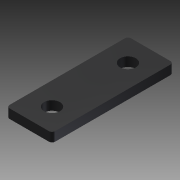
# Autodesk Inventor part: D-023
Saved by Autodesk Inventor 2015 (Build 190159000, 159)
## iProperties
Company: MARCHA TECHNOLOGY
Created: 2014-01-21
Part Number: D-023
Project: WITBOXprinter_K01
Description: SUPLEMENTO BISAGRA
Document SubType Name: Modeling
Designer: O.Martin
Stock Number: 2014000004
Density: 7.85 g/cm^3
Mass: 13.1095 g
Surface Area: 15.362 cm^2
Volume: 1.67 cm^3
Material: Steel
Appearance: Rubber - Black - Version 1.1
Author: O.Martin
Autodesk Inventor part; units mm, degrees
ref_plane "YZ Plane" through (0, 0, 0) normal (1, 0, 0) x (0, 1, 0)
ref_plane "XZ Plane" through (0, 0, 0) normal (0, 1, 0) x (-1, 0, 0)
ref_plane "XY Plane" through (0, 0, 0) normal (0, 0, 1) x (1, 0, 0)
sketch "Boceto1" plane through (0, 0, 0) normal (0, 0, 1) x (1, 0, 0)
  line L0 (-34.1303, -128.7608) -> (-49.1303, -128.7608)
  line L1 (-49.1303, -128.7608) -> (-49.1303, -88.7608)
  line L2 (-49.1303, -88.7608) -> (-34.1303, -88.7608)
  line L3 (-34.1303, -88.7608) -> (-34.1303, -128.7608)
  line L4 (-41.6303, -121.2608) -> (-41.6303, -96.2608) construction
  circle A0 centre (-41.6303, -121.2608) radius 2.6
  circle A1 centre (-41.6303, -96.2608) radius 2.6
  point P0 (-41.6303, -108.7608)
  point P1 (-34.1303, -108.7608)
  point P2 (-41.6303, -128.7608)
  dimension "d0" = 40
  dimension "d1" = 15
  dimension "d2" = 25
  dimension "d3" = 5.2
  constraints: 10 end point, 3 midpoint, 3 parallel, 2 centre point, 2 coincident, 1 equal radius, 1 horizontal, 1 horizontal alignment, 1 perpendicular, 1 vertical alignment
  measures "d0" distance of L2.end L0.start
  measures "d1" distance of L0.start L0.end
  measures "d2" distance of L4.start L4.end
  measures "d3" diameter of A0
extrude "Extrusión1" add sketch "Boceto1" along normal blind 3
fillet "Empalme1" radius 1 4 edges at (-49.1303, -128.7608, 1.5) (-34.1303, -128.7608, 1.5) (-34.1303, -88.7608, 1.5) (-49.1303, -88.7608, 1.5)
body "Solid1"
